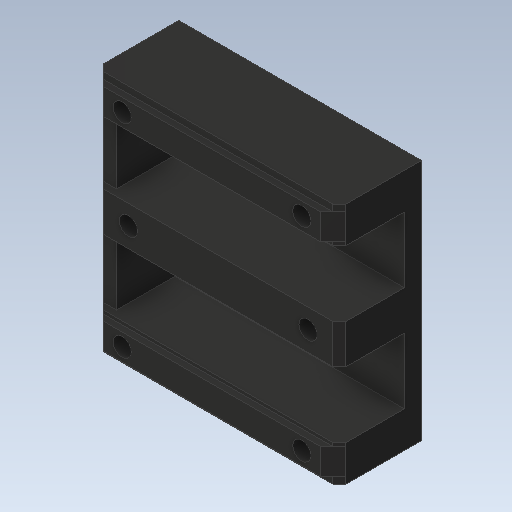
# Autodesk Inventor part: ZY_mount
Saved by Autodesk Inventor 2020 (Build 240168000, 168)
## iProperties
Created: 2020-08-11
Part Number: ZY_mount
Material: Tworzywo sztuczne PET
Document SubType Name: Modeling
Designer: invin
Density: 1.541 g/cm^3
Appearance: Kauczuk — czarny
Mass: 122.208 g
Surface Area: 266.448 cm^2
Volume: 79.3041 cm^3
Author: invin
Autodesk Inventor part; units mm, degrees
ref_plane "YZ Plane" through (0, 0, 0) normal (1, 0, 0) x (0, 1, 0)
ref_plane "XZ Plane" through (0, 0, 0) normal (0, 1, 0) x (-1, 0, 0)
ref_plane "XY Plane" through (0, 0, 0) normal (0, 0, 1) x (1, 0, 0)
sketch "Szkic1" plane through (0, 0, 0) normal (0, 0, 1) x (1, 0, 0)
  line L0 (0, 0) -> (74, 0)
  line L1 (74, 0) -> (74, 74)
  line L2 (74, 74) -> (0, 74)
  line L3 (0, 74) -> (0, 0)
  dimension "d0" = 74
  dimension "d1" = 74
  constraints: 8 end point, 2 parallel, 1 horizontal, 1 perpendicular
  measures "d0" distance of L1.end L2.end
  measures "d1" distance of L2.end L0.start
extrude "Wyciągnięcie proste1" add sketch "Szkic1" along normal blind 25
sketch "Szkic2" plane through (0, 0, 25) normal (0, 0, 1) x (1, 0, 0)
  line L0 (-55.7627, 31) -> (170, 31)
  line L1 (170, 31) -> (170, 11)
  line L2 (170, 11) -> (-55.7627, 11)
  line L3 (-55.7627, 11) -> (-55.7627, 31)
  line L4 (-31.3559, 63) -> (141.1864, 63)
  line L5 (141.1864, 63) -> (141.1864, 43)
  line L6 (141.1864, 43) -> (-31.3559, 43)
  line L7 (-31.3559, 43) -> (-31.3559, 63)
  line L8 (0, 0) -> (74, 0) projected
  line L9 (74, 74) -> (0, 74) projected
  dimension "d4" = 20
  dimension "d6" = 20
  dimension "d7" = 11
  dimension "d8" = 11
  constraints: 16 end point, 4 parallel, 2 horizontal, 2 perpendicular
  measures "d4" distance between parallel lines of L4 L6
  measures "d6" distance between parallel lines of L2 L0
  measures "d7" distance between parallel lines of L8 L2
  measures "d8" distance between parallel lines of L9 L4
extrude "Wyciągnięcie proste2" cut sketch "Szkic2" against normal blind 19.8
sketch "Szkic3" plane through (0, 0, 25) normal (0, 0, 1) x (1, 0, 0)
  line L0 (0, 9.95) -> (74, 9.95)
  line L1 (74, 9.95) -> (74, 2.05)
  line L2 (74, 2.05) -> (0, 2.05)
  line L3 (0, 2.05) -> (0, 9.95)
  line L4 (0, 71.95) -> (74, 71.95)
  line L5 (74, 71.95) -> (74, 64.05)
  line L6 (74, 64.05) -> (0, 64.05)
  line L7 (0, 64.05) -> (0, 71.95)
  line L8 (74, 74) -> (0, 74) projected
  line L9 (0, 74) -> (0, 63) projected
  line L10 (74, 63) -> (74, 74) projected
  line L11 (0, 0) -> (74, 0) projected
  line L12 (0, 11) -> (0, 0) projected
  line L13 (74, 0) -> (74, 11) projected
  dimension "d11" = 2.05
  dimension "d12" = 7.9
  dimension "d13" = 0
  dimension "d14" = 0
  dimension "d15" = 2.05
  dimension "d16" = 7.9
  dimension "d17" = 0
  dimension "d18" = 0
  constraints: 16 end point, 4 parallel, 2 horizontal, 2 perpendicular
  measures "d11" distance between parallel lines of L8 L4
  measures "d12" distance between parallel lines of L4 L6
  measures "d13" distance between parallel lines of L9 L7
  measures "d14" distance between parallel lines of L10 L5
  measures "d15" distance between parallel lines of L11 L2
  measures "d16" distance between parallel lines of L2 L0
  measures "d17" distance between parallel lines of L12 L3
  measures "d18" distance between parallel lines of L13 L1
extrude "Wyciągnięcie proste3" add sketch "Szkic3" along normal blind 1.9 contours L0 L1 L2 L3 | L4 L5 L6 L7
ref_plane "Płaszczyzna konstrukcyjna1" through (37, 0, 0) normal (1, 0, 0) x (0, 0, -1)
sketch "Szkic5" plane through (0, 0, 26.9) normal (0, 0, 1) x (1, 0, 0)
  circle A0 centre (9.61, 6) radius 2.75
  circle A1 centre (64.39, 6) radius 2.75
  line L0 (0, 0) -> (74, 0) projected
  line L1 (37, 88.8) -> (37, -14.8) projected
  dimension "d23" = 5.5
  dimension "d24" = 5.5
  dimension "d25" = 6
  dimension "d26" = 6
  dimension "d27" = 54.78
  dimension "d29" = 27.39
  constraints: 2 centre point
  measures "d23" diameter of A0
  measures "d24" diameter of A1
  measures "d25" distance from line of L0 A1.centre
  measures "d26" distance from line of L0 A0.centre
  measures "d27" distance of A1.centre A0.centre
  measures "d29" distance from line of L1 A0.centre
extrude "Wyciągnięcie proste5" cut sketch "Szkic5" against normal blind 50
pattern_linear "Szyk prostokątny1" count 3 spacing 31 along (0, 1, 0) of "Wyciągnięcie proste5"
chamfer "Faza1" distance 2 angle 45 10 edges at (0, 63.525, 25) (0, 72.975, 25) (0, 1.025, 25) (0, 10.475, 25) (0, 37, 25) (74, 1.025, 25) (74, 10.475, 25) (74, 37, 25) (74, 63.525, 25) (74, 72.975, 25)
chamfer "Faza2" distance 3.8999 angle 45 2 edges at (0, 6, 26.9) (0, 68, 26.9)
chamfer "Faza3" distance 3.8999 angle 45 2 edges at (74, 6, 26.9) (74, 68, 26.9)
sketch "Szkic6" plane through (0, 0, 0) normal (-1, 0, 0) x (0, 0, 1)
  line L0 (0, 74) -> (0, 0) projected
  line L1 (0, 0) -> (23, 0) projected
  line L2 (0, 74) -> (23, 74)
  line L3 (23, 74) -> (23, 0)
  line L4 (23, 0) -> (0, 0)
  line L5 (0, 0) -> (0, 74)
  constraints: 8 end point, 2 parallel, 1 horizontal, 1 perpendicular
extrude "Wyciągnięcie proste6" add sketch "Szkic6" against normal blind 4
